Autodesk Inventor part; units mm, degrees
(part 2 of 2)
  spline S189 degree 2 poles (-2.5096, 9.6112) (-2.4728, 9.6112) (-2.411, 9.6354) (-2.368, 9.6802) (-2.3447, 9.7402) (-2.3447, 9.7779) knots 0 0 0 1 2 3 4 4 4
  spline S190 degree 2 poles (-2.3447, 9.7779) (-2.3447, 9.8173) (-2.3716, 9.8791) (-2.4173, 9.9212) (-2.4773, 9.9436) (-2.5096, 9.9436) knots 0 0 0 1 2 3 4 4 4
  spline S191 degree 2 poles (-2.5096, 9.9436) (-2.5454, 9.9436) (-2.6072, 9.9194) (-2.6502, 9.8746) (-2.6735, 9.8146) (-2.6735, 9.7779) knots 0 0 0 1 2 3 4 4 4
  spline S192 degree 2 poles (-2.6735, 9.7779) (-2.6735, 9.7375) (-2.6458, 9.6757) (-2.6009, 9.6336) (-2.5409, 9.6112) (-2.5096, 9.6112) knots 0 0 0 1 2 3 4 4 4
  spline S193 degree 2 poles (-1.8805, 9.5709) (-1.8268, 9.5709) (-1.7766, 9.6838) (-1.7766, 9.785) knots 0 0 0 1 2 2 2
  spline S194 degree 2 poles (-1.7766, 9.785) (-1.7766, 9.8486) (-1.7999, 9.9347) (-1.8366, 9.9875) (-1.885, 10.0108) (-1.9101, 10.0108) knots 0 0 0 1 2 3 4 4 4
  spline S195 degree 2 poles (-1.9101, 10.0108) (-1.9567, 10.0108) (-2.0015, 9.9347) (-2.0051, 9.8558) knots 0 0 0 1 2 2 2
  line L242 (-2.0051, 9.8558) -> (-2.0122, 9.6551)
  spline S196 degree 2 poles (-2.0122, 9.6551) (-1.9952, 9.63) (-1.963, 9.5969) (-1.9307, 9.5789) (-1.8975, 9.5709) (-1.8805, 9.5709) knots 0 0 0 1 2 3 4 4 4
  spline S197 degree 2 poles (-2.655, 11.9876) (-2.5726, 11.9876) (-2.4382, 11.9411) (-2.3441, 11.8505) (-2.293, 11.7197) (-2.293, 11.6346) knots 0 0 0 1 2 3 4 4 4
  spline S198 degree 2 poles (-2.293, 11.6346) (-2.293, 11.5414) (-2.3423, 11.4115) (-2.4319, 11.3299) (-2.5564, 11.2923) (-2.6344, 11.2923) knots 0 0 0 1 2 3 4 4 4
  line L243 (-2.6344, 11.2923) -> (-3.3064, 11.2923)
  line L244 (-3.3064, 11.2923) -> (-3.3064, 11.4285)
  line L245 (-3.3064, 11.4285) -> (-2.6451, 11.4285)
  spline S199 degree 2 poles (-2.6451, 11.4285) (-2.586, 11.4285) (-2.4973, 11.4509) (-2.4373, 11.5011) (-2.4068, 11.5817) (-2.4068, 11.64) knots 0 0 0 1 2 3 4 4 4
  spline S200 degree 2 poles (-2.4068, 11.64) (-2.4068, 11.7484) (-2.5322, 11.8514) (-2.646, 11.8514) knots 0 0 0 1 2 2 2
  line L246 (-2.646, 11.8514) -> (-3.3064, 11.8514)
  line L247 (-3.3064, 11.8514) -> (-3.3064, 11.9876)
  line L248 (-3.3064, 11.9876) -> (-2.655, 11.9876)
  spline S201 degree 2 poles (-2.5779, 12.8335) (-2.5063, 12.8335) (-2.3996, 12.7753) (-2.3279, 12.6713) (-2.293, 12.5253) (-2.293, 12.4366) knots 0 0 0 1 2 3 4 4 4
  spline S202 degree 2 poles (-2.293, 12.4366) (-2.293, 12.3971) (-2.2993, 12.3183) (-2.3082, 12.2457) (-2.3199, 12.1812) (-2.327, 12.1552) knots 0 0 0 1 2 3 4 4 4
  line L249 (-2.327, 12.1552) -> (-2.4588, 12.1552)
  spline S203 degree 2 poles (-2.4588, 12.1552) (-2.4373, 12.2126) (-2.4131, 12.3559) (-2.4131, 12.4464) knots 0 0 0 1 2 2 2
  spline S204 degree 2 poles (-2.4131, 12.4464) (-2.4131, 12.5127) (-2.4337, 12.605) (-2.474, 12.6642) (-2.5322, 12.6911) (-2.5699, 12.6911) knots 0 0 0 1 2 3 4 4 4
  spline S205 degree 2 poles (-2.5699, 12.6911) (-2.6102, 12.6911) (-2.6675, 12.6462) (-2.7132, 12.5728) (-2.7509, 12.4787) (-2.7903, 12.3801) (-2.8369, 12.286) (-2.9005, 12.2126) (-2.9865, 12.1678) (-3.0457, 12.1678) knots 0 0 0 1 2 3 4 5 6 7 8 8 8
  spline S206 degree 2 poles (-3.0457, 12.1678) (-3.0968, 12.1678) (-3.1962, 12.2108) (-3.2733, 12.3013) (-3.3208, 12.4419) (-3.3208, 12.5405) knots 0 0 0 1 2 3 4 4 4
  spline S207 degree 2 poles (-3.3208, 12.5405) (-3.3208, 12.5656) (-3.3163, 12.6247) (-3.3082, 12.6848) (-3.2975, 12.7439) (-3.2912, 12.769) knots 0 0 0 1 2 3 4 4 4
  line L250 (-3.2912, 12.769) -> (-3.1684, 12.769)
  spline S208 degree 2 poles (-3.1684, 12.769) (-3.1855, 12.7099) (-3.2025, 12.5925) (-3.2025, 12.5369) knots 0 0 0 1 2 2 2
  spline S209 degree 2 poles (-3.2025, 12.5369) (-3.2025, 12.4204) (-3.1245, 12.3102) (-3.0591, 12.3102) knots 0 0 0 1 2 2 2
  spline S210 degree 2 poles (-3.0591, 12.3102) (-3.0188, 12.3102) (-2.9606, 12.355) (-2.914, 12.4285) (-2.8772, 12.5226) (-2.8369, 12.6212) (-2.7894, 12.7152) (-2.7249, 12.7887) (-2.6371, 12.8335) (-2.5779, 12.8335) knots 0 0 0 1 2 3 4 5 6 7 8 8 8
  spline S211 degree 2 poles (-2.6057, 13.7018) (-2.5331, 13.7018) (-2.4229, 13.6462) (-2.3459, 13.545) (-2.3064, 13.4007) (-2.3064, 13.312) knots 0 0 0 1 2 3 4 4 4
  line L251 (-2.3064, 13.312) -> (-2.3064, 13.054)
  line L252 (-2.3064, 13.054) -> (-3.3064, 13.054)
  line L253 (-3.3064, 13.054) -> (-3.3064, 13.3362)
  spline S212 degree 2 poles (-3.3064, 13.3362) (-3.3064, 13.666) (-3.0627, 13.666) knots 0 0 0 1 1 1
  spline S213 degree 2 poles (-3.0627, 13.666) (-2.9821, 13.666) (-2.8656, 13.5898) (-2.8369, 13.5038) knots 0 0 0 1 2 2 2
  spline S214 degree 2 poles (-2.8369, 13.5038) (-2.8297, 13.5441) (-2.793, 13.6158) (-2.7348, 13.6704) (-2.655, 13.7018) (-2.6057, 13.7018) knots 0 0 0 1 2 3 4 4 4
  spline S215 degree 2 poles (-2.6012, 13.5656) (-2.6389, 13.5656) (-2.6998, 13.5333) (-2.7419, 13.4724) (-2.7652, 13.3846) (-2.7652, 13.329) knots 0 0 0 1 2 3 4 4 4
  line L254 (-2.7652, 13.329) -> (-2.7652, 13.1902)
  line L255 (-2.7652, 13.1902) -> (-2.4211, 13.1902)
  line L256 (-2.4211, 13.1902) -> (-2.4211, 13.3335)
  spline S216 degree 2 poles (-2.4211, 13.3335) (-2.4211, 13.4509) (-2.508, 13.5656) (-2.6012, 13.5656) knots 0 0 0 1 2 2 2
  spline S217 degree 2 poles (-3.0448, 13.5298) (-3.0753, 13.5298) (-3.1299, 13.5118) (-3.1684, 13.4661) (-3.1917, 13.3891) (-3.1917, 13.3299) knots 0 0 0 1 2 3 4 4 4
  line L257 (-3.1917, 13.3299) -> (-3.1917, 13.1902)
  line L258 (-3.1917, 13.1902) -> (-2.8781, 13.1902)
  line L259 (-2.8781, 13.1902) -> (-2.8781, 13.3255)
  spline S218 degree 2 poles (-2.8781, 13.3255) (-2.8781, 13.3712) (-2.8978, 13.4464) (-2.9391, 13.5002) (-3.0018, 13.5298) (-3.0448, 13.5298) knots 0 0 0 1 2 3 4 4 4
  spline S219 degree 2 poles (-2.5599, 15.0982) (-2.4873, 15.0982) (-2.3771, 15.0427) (-2.3, 14.9414) (-2.2606, 14.7972) (-2.2606, 14.7084) knots 0 0 0 1 2 3 4 4 4
  line L260 (-2.2606, 14.7084) -> (-2.2606, 14.4504)
  line L261 (-2.2606, 14.4504) -> (-3.2606, 14.4504)
  line L262 (-3.2606, 14.4504) -> (-3.2606, 14.7326)
  spline S220 degree 2 poles (-3.2606, 14.7326) (-3.2606, 15.0624) (-3.0169, 15.0624) knots 0 0 0 1 1 1
  spline S221 degree 2 poles (-3.0169, 15.0624) (-2.9362, 15.0624) (-2.8197, 14.9862) (-2.791, 14.9002) knots 0 0 0 1 2 2 2
  spline S222 degree 2 poles (-2.791, 14.9002) (-2.7839, 14.9405) (-2.7471, 15.0122) (-2.6889, 15.0669) (-2.6091, 15.0982) (-2.5599, 15.0982) knots 0 0 0 1 2 3 4 4 4
  spline S223 degree 2 poles (-2.5554, 14.962) (-2.593, 14.962) (-2.6539, 14.9298) (-2.6961, 14.8688) (-2.7194, 14.781) (-2.7194, 14.7255) knots 0 0 0 1 2 3 4 4 4
  line L263 (-2.7194, 14.7255) -> (-2.7194, 14.5866)
  line L264 (-2.7194, 14.5866) -> (-2.3753, 14.5866)
  line L265 (-2.3753, 14.5866) -> (-2.3753, 14.73)
  spline S224 degree 2 poles (-2.3753, 14.73) (-2.3753, 14.8473) (-2.4622, 14.962) (-2.5554, 14.962) knots 0 0 0 1 2 2 2
  spline S225 degree 2 poles (-2.9989, 14.9262) (-3.0294, 14.9262) (-3.0841, 14.9083) (-3.1226, 14.8626) (-3.1459, 14.7855) (-3.1459, 14.7264) knots 0 0 0 1 2 3 4 4 4
  line L266 (-3.1459, 14.7264) -> (-3.1459, 14.5866)
  line L267 (-3.1459, 14.5866) -> (-2.8323, 14.5866)
  line L268 (-2.8323, 14.5866) -> (-2.8323, 14.7219)
  spline S226 degree 2 poles (-2.8323, 14.7219) (-2.8323, 14.7676) (-2.852, 14.8429) (-2.8932, 14.8966) (-2.9559, 14.9262) (-2.9989, 14.9262) knots 0 0 0 1 2 3 4 4 4
  line L269 (-2.2606, 15.8079) -> (-2.3636, 15.8052)
  spline S227 degree 2 poles (-2.3636, 15.8052) (-2.3018, 15.7425) (-2.2471, 15.6126) (-2.2471, 15.5418) knots 0 0 0 1 2 2 2
  spline S228 degree 2 poles (-2.2471, 15.5418) (-2.2471, 15.4755) (-2.2812, 15.3823) (-2.3394, 15.3222) (-2.4192, 15.2936) (-2.4658, 15.2936) knots 0 0 0 1 2 3 4 4 4
  spline S229 degree 2 poles (-2.4658, 15.2936) (-2.5814, 15.2936) (-2.7122, 15.4656) (-2.7122, 15.6341) knots 0 0 0 1 2 2 2
  line L270 (-2.7122, 15.6341) -> (-2.7122, 15.7936)
  line L271 (-2.7122, 15.7936) -> (-2.7794, 15.7936)
  spline S230 degree 2 poles (-2.7794, 15.7936) (-2.8475, 15.7936) (-2.9299, 15.7067) (-2.9299, 15.617) knots 0 0 0 1 2 2 2
  spline S231 degree 2 poles (-2.9299, 15.617) (-2.9299, 15.5516) (-2.9013, 15.4253) (-2.8744, 15.3581) knots 0 0 0 1 2 2 2
  line L272 (-2.8744, 15.3581) -> (-2.9945, 15.3581)
  spline S232 degree 2 poles (-2.9945, 15.3581) (-3.0034, 15.3832) (-3.0213, 15.445) (-3.0348, 15.514) (-3.0428, 15.5893) (-3.0428, 15.6269) knots 0 0 0 1 2 3 4 4 4
  spline S233 degree 2 poles (-3.0428, 15.6269) (-3.0428, 15.6968) (-3.0124, 15.8088) (-2.9496, 15.8859) (-2.8547, 15.9271) (-2.7901, 15.9271) knots 0 0 0 1 2 3 4 4 4
  line L273 (-2.7901, 15.9271) -> (-2.2606, 15.9271)
  line L274 (-2.2606, 15.9271) -> (-2.2606, 15.8079)
  line L275 (-2.61, 15.7936) -> (-2.61, 15.6242)
  spline S234 degree 2 poles (-2.61, 15.6242) (-2.61, 15.574) (-2.5903, 15.5024) (-2.5536, 15.4567) (-2.5025, 15.4343) (-2.4703, 15.4343) knots 0 0 0 1 2 3 4 4 4
  spline S235 degree 2 poles (-2.4703, 15.4343) (-2.4479, 15.4343) (-2.4075, 15.4477) (-2.3762, 15.4791) (-2.3582, 15.5274) (-2.3582, 15.5633) knots 0 0 0 1 2 3 4 4 4
  spline S236 degree 2 poles (-2.3582, 15.5633) (-2.3582, 15.609) (-2.4138, 15.7273) (-2.4738, 15.7936) knots 0 0 0 1 2 2 2
  line L276 (-2.4738, 15.7936) -> (-2.61, 15.7936)
  spline S237 degree 2 poles (-2.2713, 16.7954) (-2.2597, 16.7506) (-2.2498, 16.6538) (-2.2498, 16.6036) knots 0 0 0 1 2 2 2
  spline S238 degree 2 poles (-2.2498, 16.6036) (-2.2498, 16.4593) (-2.3807, 16.3169) (-2.516, 16.3169) knots 0 0 0 1 2 2 2
  line L277 (-2.516, 16.3169) -> (-2.9165, 16.3169)
  line L278 (-2.9165, 16.3169) -> (-2.9165, 16.1018)
  line L279 (-2.9165, 16.1018) -> (-3.0285, 16.1018)
  line L280 (-3.0285, 16.1018) -> (-3.0285, 16.3169)
  line L281 (-3.0285, 16.3169) -> (-3.24, 16.3169)
  line L282 (-3.24, 16.3169) -> (-3.274, 16.4504)
  line L283 (-3.274, 16.4504) -> (-3.0285, 16.4504)
  line L284 (-3.0285, 16.4504) -> (-3.0285, 16.7954)
  line L285 (-3.0285, 16.7954) -> (-2.9165, 16.7954)
  line L286 (-2.9165, 16.7954) -> (-2.9165, 16.4504)
  line L287 (-2.9165, 16.4504) -> (-2.5267, 16.4504)
  spline S239 degree 2 poles (-2.5267, 16.4504) (-2.4443, 16.4504) (-2.3627, 16.5382) (-2.3627, 16.6242) knots 0 0 0 1 2 2 2
  spline S240 degree 2 poles (-2.3627, 16.6242) (-2.3627, 16.661) (-2.3744, 16.7479) (-2.386, 16.7954) knots 0 0 0 1 2 2 2
  line L288 (-2.386, 16.7954) -> (-2.2713, 16.7954)
  line L289 (-3.2305, 18.0782) -> (-2.2305, 17.7377)
  line L290 (-2.2305, 17.7377) -> (-2.2305, 17.554)
  line L291 (-2.2305, 17.554) -> (-3.2305, 17.2225)
  line L292 (-3.2305, 17.2225) -> (-3.2305, 17.3757)
  line L293 (-3.2305, 17.3757) -> (-2.5567, 17.5917)
  line L294 (-2.5567, 17.5917) -> (-2.3587, 17.6535)
  line L295 (-2.3587, 17.6535) -> (-2.5567, 17.7162)
  line L296 (-2.5567, 17.7162) -> (-3.2305, 17.9322)
  line L297 (-3.2305, 17.9322) -> (-3.2305, 18.0782)
  spline S241 degree 2 poles (-2.4402, 18.8112) (-2.3999, 18.8112) (-2.3354, 18.7834) (-2.2861, 18.7359) (-2.2512, 18.6732) (-2.2279, 18.6024) (-2.2171, 18.5271) (-2.2171, 18.4913) knots 0 0 0 1 2 3 4 5 6 6 6
  spline S242 degree 2 poles (-2.2171, 18.4913) (-2.2171, 18.4133) (-2.2314, 18.2825) (-2.2467, 18.2198) knots 0 0 0 1 2 2 2
  line L298 (-2.2467, 18.2198) -> (-2.3694, 18.2198)
  spline S243 degree 2 poles (-2.3694, 18.2198) (-2.3497, 18.287) (-2.33, 18.4205) (-2.33, 18.4859) knots 0 0 0 1 2 2 2
  spline S244 degree 2 poles (-2.33, 18.4859) (-2.33, 18.5818) (-2.382, 18.6732) (-2.4295, 18.6732) knots 0 0 0 1 2 2 2
  spline S245 degree 2 poles (-2.4295, 18.6732) (-2.4501, 18.6732) (-2.4832, 18.6589) (-2.5128, 18.6203) (-2.5451, 18.5406) (-2.5657, 18.4707) knots 0 0 0 1 2 3 4 4 4
  spline S246 degree 2 poles (-2.5657, 18.4707) (-2.5809, 18.4187) (-2.6203, 18.3309) (-2.6741, 18.2664) (-2.7458, 18.2297) (-2.7951, 18.2297) knots 0 0 0 1 2 3 4 4 4
  spline S247 degree 2 poles (-2.7951, 18.2297) (-2.8273, 18.2297) (-2.9035, 18.2592) (-2.9689, 18.3318) (-3.0128, 18.4537) (-3.0128, 18.546) knots 0 0 0 1 2 3 4 4 4
  spline S248 degree 2 poles (-3.0128, 18.546) (-3.0128, 18.5908) (-3.0029, 18.701) (-2.9904, 18.761) knots 0 0 0 1 2 2 2
  line L299 (-2.9904, 18.761) -> (-2.8721, 18.761)
  spline S249 degree 2 poles (-2.8721, 18.761) (-2.8874, 18.6983) (-2.9017, 18.5854) (-2.9017, 18.5442) knots 0 0 0 1 2 2 2
  spline S250 degree 2 poles (-2.9017, 18.5442) (-2.9017, 18.4949) (-2.8865, 18.4268) (-2.8596, 18.3847) (-2.8237, 18.3659) (-2.8031, 18.3659) knots 0 0 0 1 2 3 4 4 4
  spline S251 degree 2 poles (-2.8031, 18.3659) (-2.7825, 18.3659) (-2.7485, 18.382) (-2.7171, 18.4259) (-2.6857, 18.5038) (-2.6678, 18.5666) knots 0 0 0 1 2 3 4 4 4
  spline S252 degree 2 poles (-2.6678, 18.5666) (-2.6481, 18.6347) (-2.6042, 18.7279) (-2.5504, 18.7861) (-2.4832, 18.8112) (-2.4402, 18.8112) knots 0 0 0 1 2 3 4 4 4
  line L300 (-2.274, 20.422) -> (-2.274, 19.853)
  line L301 (-2.274, 19.853) -> (-3.274, 19.853)
  line L302 (-3.274, 19.853) -> (-3.274, 20.422)
  line L303 (-3.274, 20.422) -> (-3.1593, 20.422)
  line L304 (-3.1593, 20.422) -> (-3.1593, 19.9892)
  line L305 (-3.1593, 19.9892) -> (-2.8493, 19.9892)
  line L306 (-2.8493, 19.9892) -> (-2.8493, 20.405)
  line L307 (-2.8493, 20.405) -> (-2.7346, 20.405)
  line L308 (-2.7346, 20.405) -> (-2.7346, 19.9892)
  line L309 (-2.7346, 19.9892) -> (-2.3905, 19.9892)
  line L310 (-2.3905, 19.9892) -> (-2.3905, 20.422)
  line L311 (-2.3905, 20.422) -> (-2.274, 20.422)
  line L312 (-2.274, 21.3324) -> (-2.274, 21.1478)
  line L313 (-2.274, 21.1478) -> (-2.8977, 20.8691)
  line L314 (-2.8977, 20.8691) -> (-3.0984, 20.7885)
  line L315 (-3.0984, 20.7885) -> (-2.5939, 20.7885)
  line L316 (-2.5939, 20.7885) -> (-2.274, 20.7885)
  line L317 (-2.274, 20.7885) -> (-2.274, 20.6523)
  line L318 (-2.274, 20.6523) -> (-3.274, 20.6523)
  line L319 (-3.274, 20.6523) -> (-3.274, 20.8342)
  line L320 (-3.274, 20.8342) -> (-2.6826, 21.1003)
  line L321 (-2.6826, 21.1003) -> (-2.4541, 21.1962)
  line L322 (-2.4541, 21.1962) -> (-2.99, 21.1962)
  line L323 (-2.99, 21.1962) -> (-3.274, 21.1962)
  line L324 (-3.274, 21.1962) -> (-3.274, 21.3324)
  line L325 (-3.274, 21.3324) -> (-2.274, 21.3324)
  spline S253 degree 2 poles (-3.1163, 22.8315) (-3.1459, 22.7759) (-3.179, 22.6576) (-3.179, 22.5877) knots 0 0 0 1 2 2 2
  spline S254 degree 2 poles (-3.179, 22.5877) (-3.179, 22.5089) (-3.1226, 22.3843) (-3.0195, 22.2992) (-2.8735, 22.2544) (-2.7857, 22.2544) knots 0 0 0 1 2 3 4 4 4
  spline S255 degree 2 poles (-2.7857, 22.2544) (-2.6943, 22.2544) (-2.5482, 22.2911) (-2.4479, 22.3691) (-2.3941, 22.491) (-2.3941, 22.5761) knots 0 0 0 1 2 3 4 4 4
  spline S256 degree 2 poles (-2.3941, 22.5761) (-2.3941, 22.5904) (-2.3968, 22.6245) (-2.4022, 22.6576) (-2.4102, 22.689) (-2.4147, 22.7015) knots 0 0 0 1 2 3 4 4 4
  line L326 (-2.4147, 22.7015) -> (-2.7328, 22.7015)
  line L327 (-2.7328, 22.7015) -> (-2.7328, 22.4972)
  line L328 (-2.7328, 22.4972) -> (-2.8457, 22.4972)
  line L329 (-2.8457, 22.4972) -> (-2.8457, 22.8359)
  line L330 (-2.8457, 22.8359) -> (-2.3341, 22.8359)
  spline S257 degree 2 poles (-2.3341, 22.8359) (-2.3197, 22.8046) (-2.2973, 22.7347) (-2.2821, 22.6621) (-2.274, 22.5904) (-2.274, 22.5564) knots 0 0 0 1 2 3 4 4 4
  spline S258 degree 2 poles (-2.274, 22.5564) (-2.274, 22.4542) (-2.3385, 22.2893) (-2.4649, 22.1738) (-2.6531, 22.1119) (-2.7767, 22.1119) knots 0 0 0 1 2 3 4 4 4
  spline S259 degree 2 poles (-2.7767, 22.1119) (-2.9004, 22.1119) (-3.0948, 22.1809) (-3.231, 22.3055) (-3.3018, 22.4811) (-3.3018, 22.5868) knots 0 0 0 1 2 3 4 4 4
  spline S260 degree 2 poles (-3.3018, 22.5868) (-3.3018, 22.654) (-3.2776, 22.7759) (-3.2516, 22.8315) knots 0 0 0 1 2 2 2
  line L331 (-3.2516, 22.8315) -> (-3.1163, 22.8315)
  line L332 (-2.2875, 23.6953) -> (-2.2875, 23.5107)
  line L333 (-2.2875, 23.5107) -> (-2.9111, 23.232)
  line L334 (-2.9111, 23.232) -> (-3.1118, 23.1514)
  line L335 (-3.1118, 23.1514) -> (-2.6074, 23.1514)
  line L336 (-2.6074, 23.1514) -> (-2.2875, 23.1514)
  line L337 (-2.2875, 23.1514) -> (-2.2875, 23.0152)
  line L338 (-2.2875, 23.0152) -> (-3.2875, 23.0152)
  line L339 (-3.2875, 23.0152) -> (-3.2875, 23.1971)
  line L340 (-3.2875, 23.1971) -> (-2.6961, 23.4632)
  line L341 (-2.6961, 23.4632) -> (-2.4676, 23.5591)
  line L342 (-2.4676, 23.5591) -> (-3.0034, 23.5591)
  line L343 (-3.0034, 23.5591) -> (-3.2875, 23.5591)
  line L344 (-3.2875, 23.5591) -> (-3.2875, 23.6953)
  line L345 (-3.2875, 23.6953) -> (-2.2875, 23.6953)
  spline S261 degree 2 poles (-2.7982, 24.5913) (-2.7265, 24.5913) (-2.5948, 24.5689) (-2.4819, 24.5205) (-2.3896, 24.4426) (-2.3233, 24.3288) (-2.2875, 24.1791) (-2.2875, 24.0833) knots 0 0 0 1 2 3 4 5 6 6 6
  line L346 (-2.2875, 24.0833) -> (-2.2875, 23.8691)
  line L347 (-2.2875, 23.8691) -> (-3.2875, 23.8691)
  line L348 (-3.2875, 23.8691) -> (-3.2875, 24.1272)
  spline S262 degree 2 poles (-3.2875, 24.1272) (-3.2875, 24.361) (-3.0464, 24.5913) (-2.7982, 24.5913) knots 0 0 0 1 2 2 2
  spline S263 degree 2 poles (-2.7893, 24.448) (-2.895, 24.448) (-3.0419, 24.4085) (-3.1324, 24.327) (-3.1728, 24.2051) (-3.1728, 24.1227) knots 0 0 0 1 2 3 4 4 4
  line L349 (-3.1728, 24.1227) -> (-3.1728, 24.0053)
  line L350 (-3.1728, 24.0053) -> (-2.4057, 24.0053)
  line L351 (-2.4057, 24.0053) -> (-2.4057, 24.1066)
  spline S264 degree 2 poles (-2.4057, 24.1066) (-2.4057, 24.448) (-2.7893, 24.448) knots 0 0 0 1 1 1
  spline S265 degree 2 poles (-3.1922, 28.5235) (-3.2218, 28.4679) (-3.2549, 28.3496) (-3.2549, 28.2798) knots 0 0 0 1 2 2 2
  spline S266 degree 2 poles (-3.2549, 28.2798) (-3.2549, 28.2009) (-3.1985, 28.0763) (-3.0954, 27.9912) (-2.9494, 27.9464) (-2.8616, 27.9464) knots 0 0 0 1 2 3 4 4 4
  spline S267 degree 2 poles (-2.8616, 27.9464) (-2.7702, 27.9464) (-2.6241, 27.9832) (-2.5237, 28.0611) (-2.47, 28.183) (-2.47, 28.2681) knots 0 0 0 1 2 3 4 4 4
  spline S268 degree 2 poles (-2.47, 28.2681) (-2.47, 28.2824) (-2.4727, 28.3165) (-2.4781, 28.3496) (-2.4861, 28.381) (-2.4906, 28.3936) knots 0 0 0 1 2 3 4 4 4
  line L352 (-2.4906, 28.3936) -> (-2.8087, 28.3936)
  line L353 (-2.8087, 28.3936) -> (-2.8087, 28.1893)
  line L354 (-2.8087, 28.1893) -> (-2.9216, 28.1893)
  line L355 (-2.9216, 28.1893) -> (-2.9216, 28.528)
  line L356 (-2.9216, 28.528) -> (-2.4099, 28.528)
  spline S269 degree 2 poles (-2.4099, 28.528) (-2.3956, 28.4966) (-2.3732, 28.4267) (-2.358, 28.3541) (-2.3499, 28.2824) (-2.3499, 28.2484) knots 0 0 0 1 2 3 4 4 4
  spline S270 degree 2 poles (-2.3499, 28.2484) (-2.3499, 28.1462) (-2.4144, 27.9814) (-2.5408, 27.8658) (-2.7289, 27.8039) (-2.8526, 27.8039) knots 0 0 0 1 2 3 4 4 4
  spline S271 degree 2 poles (-2.8526, 27.8039) (-2.9763, 27.8039) (-3.1707, 27.8729) (-3.3069, 27.9975) (-3.3777, 28.1731) (-3.3777, 28.2789) knots 0 0 0 1 2 3 4 4 4
  spline S272 degree 2 poles (-3.3777, 28.2789) (-3.3777, 28.3461) (-3.3535, 28.4679) (-3.3275, 28.5235) knots 0 0 0 1 2 2 2
  line L357 (-3.3275, 28.5235) -> (-3.1922, 28.5235)
  spline S273 degree 2 poles (-2.7022, 30.4878) (-2.6278, 30.4878) (-2.506, 30.4232) (-2.4182, 30.3112) (-2.3689, 30.158) (-2.3689, 30.0693) knots 0 0 0 1 2 3 4 4 4
  spline S274 degree 2 poles (-2.3689, 30.0693) (-2.3689, 30.0469) (-2.3716, 29.9958) (-2.3752, 29.9447) (-2.3796, 29.8964) (-2.3823, 29.8775) knots 0 0 0 1 2 3 4 4 4
  line L358 (-2.3823, 29.8775) -> (-2.5033, 29.8775)
  spline S275 degree 2 poles (-2.5033, 29.8775) (-2.4934, 29.9188) (-2.4845, 30.0254) (-2.4845, 30.0792) knots 0 0 0 1 2 2 2
  spline S276 degree 2 poles (-2.4845, 30.0792) (-2.4845, 30.141) (-2.5132, 30.2386) (-2.5678, 30.3076) (-2.6449, 30.3444) (-2.6933, 30.3444) knots 0 0 0 1 2 3 4 4 4
  spline S277 degree 2 poles (-2.6933, 30.3444) (-2.7865, 30.3444) (-2.8716, 30.2109) (-2.8716, 30.0854) knots 0 0 0 1 2 2 2
  line L359 (-2.8716, 30.0854) -> (-2.8716, 29.8955)
  line L360 (-2.8716, 29.8955) -> (-3.3823, 29.8955)
  line L361 (-3.3823, 29.8955) -> (-3.3823, 30.434)
  line L362 (-3.3823, 30.434) -> (-3.2658, 30.434)
  line L363 (-3.2658, 30.434) -> (-3.2658, 30.0209)
  line L364 (-3.2658, 30.0209) -> (-2.9854, 30.0209)
  line L365 (-2.9854, 30.0209) -> (-2.9854, 30.1078)
  spline S278 degree 2 poles (-2.9854, 30.1078) (-2.9854, 30.1804) (-2.9594, 30.3166) (-2.894, 30.4223) (-2.7847, 30.4878) (-2.7022, 30.4878) knots 0 0 0 1 2 3 4 4 4
  line L366 (-3.3823, 31.4627) -> (-2.3823, 31.1222)
  line L367 (-2.3823, 31.1222) -> (-2.3823, 30.9385)
  line L368 (-2.3823, 30.9385) -> (-3.3823, 30.6069)
  line L369 (-3.3823, 30.6069) -> (-3.3823, 30.7602)
  line L370 (-3.3823, 30.7602) -> (-2.7085, 30.9761)
  line L371 (-2.7085, 30.9761) -> (-2.5105, 31.0379)
  line L372 (-2.5105, 31.0379) -> (-2.7085, 31.1007)
  line L373 (-2.7085, 31.1007) -> (-3.3823, 31.3166)
  line L374 (-3.3823, 31.3166) -> (-3.3823, 31.4627)
  spline S279 degree 2 poles (-2.9486, 33.1319) (-2.8877, 33.1319) (-2.7676, 33.0862) (-2.6726, 32.9894) (-2.6135, 32.8398) (-2.6135, 32.735) knots 0 0 0 1 2 3 4 4 4
  line L375 (-2.6135, 32.735) -> (-2.6135, 32.6113)
  line L376 (-2.6135, 32.6113) -> (-2.255, 32.6113)
  line L377 (-2.255, 32.6113) -> (-2.255, 32.4751)
  line L378 (-2.255, 32.4751) -> (-3.255, 32.4751)
  line L379 (-3.255, 32.4751) -> (-3.255, 32.7565)
  spline S280 degree 2 poles (-3.255, 32.7565) (-3.255, 32.8308) (-3.2219, 32.967) (-3.1484, 33.071) (-3.0319, 33.1319) (-2.9486, 33.1319) knots 0 0 0 1 2 3 4 4 4
  spline S281 degree 2 poles (-2.9432, 32.9903) (-3.0391, 32.9903) (-3.1421, 32.864) (-3.1421, 32.7511) knots 0 0 0 1 2 2 2
  line L380 (-3.1421, 32.7511) -> (-3.1421, 32.6113)
  line L381 (-3.1421, 32.6113) -> (-2.73, 32.6113)
  line L382 (-2.73, 32.6113) -> (-2.73, 32.7385)
  spline S282 degree 2 poles (-2.73, 32.7385) (-2.73, 32.8595) (-2.8357, 32.9903) (-2.9432, 32.9903) knots 0 0 0 1 2 2 2
  line L383 (-3.255, 34.0432) -> (-2.255, 33.976)
  line L384 (-2.255, 33.976) -> (-2.255, 33.7995)
  line L385 (-2.255, 33.7995) -> (-2.6108, 33.6749)
  line L386 (-2.6108, 33.6749) -> (-2.7246, 33.6409)
  line L387 (-2.7246, 33.6409) -> (-2.6018, 33.605)
  line L388 (-2.6018, 33.605) -> (-2.255, 33.4894)
  line L389 (-2.255, 33.4894) -> (-2.255, 33.3192)
  line L390 (-2.255, 33.3192) -> (-3.255, 33.2502)
  line L391 (-3.255, 33.2502) -> (-3.255, 33.3783)
  line L392 (-3.255, 33.3783) -> (-2.574, 33.4178)
  line L393 (-2.574, 33.4178) -> (-2.3877, 33.4294)
  line L394 (-2.3877, 33.4294) -> (-2.5463, 33.4778)
  line L395 (-2.5463, 33.4778) -> (-2.9172, 33.5988)
  line L396 (-2.9172, 33.5988) -> (-2.9172, 33.6928)
  line L397 (-2.9172, 33.6928) -> (-2.5194, 33.8326)
  line L398 (-2.5194, 33.8326) -> (-2.3877, 33.8792)
  line L399 (-2.3877, 33.8792) -> (-2.5248, 33.8819)
  line L400 (-2.5248, 33.8819) -> (-3.255, 33.9213)
  line L401 (-3.255, 33.9213) -> (-3.255, 34.0432)
  line L402 (-2.255, 34.8828) -> (-2.255, 34.7287)
  line L403 (-2.255, 34.7287) -> (-2.5749, 34.579)
  spline S283 degree 2 poles (-2.5749, 34.579) (-2.6117, 34.5629) (-2.6601, 34.5271) (-2.6878, 34.4867) (-2.7004, 34.4384) (-2.7004, 34.4088) knots 0 0 0 1 2 3 4 4 4
  line L404 (-2.7004, 34.4088) -> (-2.7004, 34.3443)
  line L405 (-2.7004, 34.3443) -> (-2.255, 34.3443)
  line L406 (-2.255, 34.3443) -> (-2.255, 34.2081)
  line L407 (-2.255, 34.2081) -> (-3.255, 34.2081)
  line L408 (-3.255, 34.2081) -> (-3.255, 34.476)
  spline S284 degree 2 poles (-3.255, 34.476) (-3.255, 34.5629) (-3.2165, 34.6884) (-3.1475, 34.769) (-3.0507, 34.8066) (-2.9916, 34.8066) knots 0 0 0 1 2 3 4 4 4
  spline S285 degree 2 poles (-2.9916, 34.8066) (-2.945, 34.8066) (-2.8617, 34.7789) (-2.7936, 34.7251) (-2.7443, 34.6445) (-2.7317, 34.5925) knots 0 0 0 1 2 3 4 4 4
  spline S286 degree 2 poles (-2.7317, 34.5925) (-2.7174, 34.6346) (-2.6448, 34.6937) (-2.5839, 34.7242) knots 0 0 0 1 2 2 2
  line L409 (-2.5839, 34.7242) -> (-2.255, 34.8828)
  spline S287 degree 2 poles (-2.98, 34.6642) (-3.0606, 34.6642) (-3.1404, 34.5638) (-3.1404, 34.4724) knots 0 0 0 1 2 2 2
  line L410 (-3.1404, 34.4724) -> (-3.1404, 34.3443)
  line L411 (-3.1404, 34.3443) -> (-2.8097, 34.3443)
  line L412 (-2.8097, 34.3443) -> (-2.8097, 34.4545)
  spline S288 degree 2 poles (-2.8097, 34.4545) (-2.8097, 34.5029) (-2.8321, 34.5799) (-2.8751, 34.6346) (-2.9387, 34.6642) (-2.98, 34.6642) knots 0 0 0 1 2 3 4 4 4
  point P0 (0, 0)
  constraints: 24 other
extrude "Extrusión6" add sketch "textos" along normal blind 0.03 separate body
